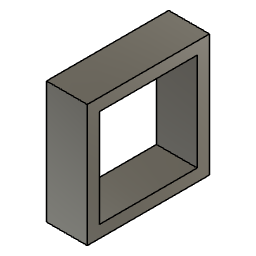
mainrod fitting v1.1 (Autodesk Fusion 360 design; units mm, degrees)
Autodesk Fusion 360 part; units mm, degrees
sketch "Sketch1" plane through (0, 0, 0) normal (1, 0, 0) x (0, 1, 0)
  line L0 (9.5131, 10.735) -> (-5.4869, 10.735)
  line L1 (-5.4869, 10.735) -> (-5.4869, -4.265)
  line L2 (-5.4869, -4.265) -> (9.5131, -4.265)
  line L3 (9.5131, -4.265) -> (9.5131, 10.735)
  line L4 (9.5131, 10.735) -> (-5.4869, -4.265) construction
  line L5 (-5.4869, 10.735) -> (9.5131, -4.265) construction
  line L6 (8.0131, -2.765) -> (-3.9869, -2.765)
  line L7 (-3.9869, -2.765) -> (-3.9869, 9.235)
  line L8 (-3.9869, 9.235) -> (8.0131, 9.235)
  line L9 (8.0131, 9.235) -> (8.0131, -2.765)
  line L10 (8.0131, -2.765) -> (-3.9869, 9.235) construction
  line L11 (-3.9869, -2.765) -> (8.0131, 9.235) construction
  point P0 (2.0131, 3.235)
  point P1 (2.0131, 3.235)
  dimension "d3" = 15
  dimension "d4" = 15
  dimension "d5" = 12
  dimension "d6" = 12
  constraint horizontal L0
  constraint perpendicular L0 L1
  constraint parallel L0 L2
  constraint parallel L1 L3
  constraint coincident L4 P1
  constraint coincident L5 P1
  constraint horizontal L6
  constraint perpendicular L6 L7
  constraint parallel L6 L8
  constraint parallel L7 L9
  constraint coincident L10 P1
  constraint coincident L11 P1
  constraint coincident P1 P0
  measures "d3" distance of L1.end L2.end
  measures "d4" distance of L0.end L1.end
  measures "d5" distance of L7.end L8.end
  measures "d6" distance of L6.end L7.end
extrude "Extrude1" add sketch "Sketch1" along normal blind 5
